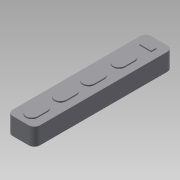
# Autodesk Inventor part: power strip
Saved by Autodesk Inventor 2015 (Build 190159000, 159)
## iProperties
Created: 2015-05-22
Part Number: power strip
Material: Generic
Document SubType Name: Modeling
Designer: Joe Sheldon
Density: 1 g/cm^3
Appearance: Default
Author: Joe Sheldon
Autodesk Inventor part; units mm, degrees
ref_plane "YZ Plane" through (0, 0, 0) normal (1, 0, 0) x (0, 1, 0)
ref_plane "XZ Plane" through (0, 0, 0) normal (0, 1, 0) x (-1, 0, 0)
ref_plane "XY Plane" through (0, 0, 0) normal (0, 0, 1) x (1, 0, 0)
sketch "Sketch1" plane through (0, 0, 0) normal (0, 1, 0) x (-1, 0, 0)
  line L0 (0, 0) -> (69.85, 0)
  line L1 (69.85, 0) -> (69.85, -355.6)
  line L2 (69.85, -355.6) -> (0, -355.6)
  line L3 (0, -355.6) -> (0, 0)
  dimension "d0" = 69.85
  dimension "d1" = 355.6
  constraints: 8 end point, 2 parallel, 1 horizontal, 1 perpendicular
  measures "d0" distance of L1.end L2.end
  measures "d1" distance of L0.end L1.end
extrude "Extrusion1" add sketch "Sketch1" along normal blind 44.45
fillet "Fillet1" radius 14.2875 4 edges at (0, 22.225, 0) (-69.85, 22.225, 0) (0, 22.225, -355.6) (-69.85, 22.225, -355.6)
sketch "Sketch2" plane through (0, 44.45, 0) normal (0, 1, 0) x (1, 0, 0)
  arc A0 (-55.5625, 355.6) -> (-69.85, 341.3125) centre (-55.5625, 341.3125) ccw projected
  line L0 (-69.85, 341.3125) -> (-69.85, 14.2875) projected
  arc A1 (-69.85, 14.2875) -> (-55.5625, 0) centre (-55.5625, 14.2875) ccw projected
  line L1 (-55.5625, 0) -> (-14.2875, 0) projected
  arc A2 (-14.2875, 0) -> (0, 14.2875) centre (-14.2875, 14.2875) ccw projected
  line L2 (0, 14.2875) -> (0, 341.3125) projected
  arc A3 (0, 341.3125) -> (-14.2875, 355.6) centre (-14.2875, 341.3125) ccw projected
  line L3 (-14.2875, 355.6) -> (-55.5625, 355.6) projected
  line L4 (-34.925, 28.5275) -> (-34.925, 53.9275) construction
  line L5 (-19.685, 28.5275) -> (-19.685, 53.9275)
  line L6 (-50.165, 53.9275) -> (-50.165, 28.5275)
  arc A4 (-50.165, 28.5275) -> (-19.685, 28.5275) centre (-34.925, 28.5275) ccw
  arc A5 (-19.685, 53.9275) -> (-50.165, 53.9275) centre (-34.925, 53.9275) ccw
  line L7 (-34.925, 102.0822) -> (-34.925, 127.4822) construction
  line L8 (-19.685, 102.0822) -> (-19.685, 127.4822)
  line L9 (-50.165, 127.4822) -> (-50.165, 102.0822)
  arc A6 (-50.165, 102.0822) -> (-19.685, 102.0822) centre (-34.925, 102.0822) ccw
  arc A7 (-19.685, 127.4822) -> (-50.165, 127.4822) centre (-34.925, 127.4822) ccw
  line L10 (-34.925, 174.3115) -> (-34.925, 199.7115) construction
  line L11 (-19.685, 174.3115) -> (-19.685, 199.7115)
  line L12 (-50.165, 199.7115) -> (-50.165, 174.3115)
  arc A8 (-50.165, 174.3115) -> (-19.685, 174.3115) centre (-34.925, 174.3115) ccw
  arc A9 (-19.685, 199.7115) -> (-50.165, 199.7115) centre (-34.925, 199.7115) ccw
  line L13 (-34.925, 252.1734) -> (-34.925, 277.5734) construction
  line L14 (-19.685, 252.1734) -> (-19.685, 277.5734)
  line L15 (-50.165, 277.5734) -> (-50.165, 252.1734)
  arc A10 (-50.165, 252.1734) -> (-19.685, 252.1734) centre (-34.925, 252.1734) ccw
  arc A11 (-19.685, 277.5734) -> (-50.165, 277.5734) centre (-34.925, 277.5734) ccw
  point P0 (0, 0)
  point P1 (-34.925, 41.2275)
  point P2 (-34.925, 114.7822)
  point P3 (-34.925, 187.0115)
  point P4 (-34.925, 264.8734)
  dimension "d5" = 25.4
  dimension "d6" = 30.48
  dimension "d7" = 25.4
  dimension "d8" = 30.48
  dimension "d9" = 25.4
  dimension "d10" = 30.48
  dimension "d11" = 25.4
  dimension "d12" = 30.48
  constraints: 32 end point, 16 point on circle, 16 tangent, 8 centre point, 6 point on line, 4 midpoint, 4 parallel, 1 vertical
  measures "d5" distance of L4.start L4.end
  measures "d6" diameter of A5
  measures "d7" distance of L7.start L7.end
  measures "d8" diameter of A7
  measures "d9" distance of L10.start L10.end
  measures "d10" diameter of A9
  measures "d11" distance of L13.start L13.end
  measures "d12" diameter of A11
extrude "Extrusion2" add sketch "Sketch2" along normal blind 3.175 contours A4 L6 A5 L5 | A6 L9 A7 L8 | A8 L12 A9 L11 | A10 L15 A11 L14
sketch "Sketch3" plane through (0, 44.45, 0) normal (0, 1, 0) x (1, 0, 0)
  arc A0 (-50.165, 174.3115) -> (-19.685, 174.3115) centre (-34.925, 174.3115) ccw projected
  line L0 (-50.165, 174.3115) -> (-50.165, 199.7115) projected
  arc A1 (-19.685, 199.7115) -> (-50.165, 199.7115) centre (-34.925, 199.7115) ccw projected
  line L1 (-19.685, 199.7115) -> (-19.685, 174.3115) projected
  arc A2 (-50.165, 28.5275) -> (-19.685, 28.5275) centre (-34.925, 28.5275) ccw projected
  line L2 (-50.165, 28.5275) -> (-50.165, 53.9275) projected
  arc A3 (-19.685, 53.9275) -> (-50.165, 53.9275) centre (-34.925, 53.9275) ccw projected
  line L3 (-19.685, 53.9275) -> (-19.685, 28.5275) projected
  arc A4 (-50.165, 102.0822) -> (-19.685, 102.0822) centre (-34.925, 102.0822) ccw projected
  line L4 (-50.165, 102.0822) -> (-50.165, 127.4822) projected
  arc A5 (-19.685, 127.4822) -> (-50.165, 127.4822) centre (-34.925, 127.4822) ccw projected
  line L5 (-19.685, 127.4822) -> (-19.685, 102.0822) projected
  arc A6 (-50.165, 252.1734) -> (-19.685, 252.1734) centre (-34.925, 252.1734) ccw projected
  line L6 (-50.165, 252.1734) -> (-50.165, 277.5734) projected
  arc A7 (-19.685, 277.5734) -> (-50.165, 277.5734) centre (-34.925, 277.5734) ccw projected
  line L7 (-19.685, 277.5734) -> (-19.685, 252.1734) projected
  arc A8 (-55.5625, 355.6) -> (-69.85, 341.3125) centre (-55.5625, 341.3125) ccw projected
  line L8 (-69.85, 341.3125) -> (-69.85, 14.2875) projected
  arc A9 (-69.85, 14.2875) -> (-55.5625, 0) centre (-55.5625, 14.2875) ccw projected
  line L9 (-55.5625, 0) -> (-14.2875, 0) projected
  arc A10 (-14.2875, 0) -> (0, 14.2875) centre (-14.2875, 14.2875) ccw projected
  line L10 (0, 14.2875) -> (0, 341.3125) projected
  arc A11 (0, 341.3125) -> (-14.2875, 355.6) centre (-14.2875, 341.3125) ccw projected
  line L11 (-14.2875, 355.6) -> (-55.5625, 355.6) projected
  line L12 (-19.685, 333.0203) -> (-50.165, 333.0203)
  line L13 (-50.165, 333.0203) -> (-50.165, 319.6698)
  line L14 (-50.165, 319.6698) -> (-19.685, 319.6698)
  line L15 (-19.685, 319.6698) -> (-19.685, 333.0203)
  line L16 (-19.685, 333.0203) -> (-50.165, 319.6698) construction
  line L17 (-50.165, 333.0203) -> (-19.685, 319.6698) construction
  point P0 (0, 0)
  point P1 (-34.925, 326.345)
  constraints: 12 end point, 2 midpoint, 2 parallel, 1 horizontal, 1 perpendicular
extrude "Extrusion3" add sketch "Sketch3" along normal blind 3.175 contours L15 L14 L13 L12
body "Solid1"
